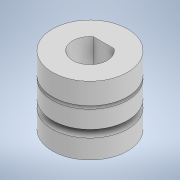
# Autodesk Inventor part: V-Groove Feeder
Saved by Autodesk Inventor 2022.2 (Build 262287000, 287)
## iProperties
Created: 2022-08-20
Part Number: V-Groove Feeder
Material: Generic
Document SubType Name: Modeling
Designer: Ilewicz
Density: 1 g/cm^3
Appearance: Default
Author: Ilewicz
Autodesk Inventor part; units mm, degrees
ref_plane "YZ Plane" through (0, 0, 0) normal (1, 0, 0) x (0, 1, 0)
ref_plane "XZ Plane" through (0, 0, 0) normal (0, 1, 0) x (-1, 0, 0)
ref_plane "XY Plane" through (0, 0, 0) normal (0, 0, 1) x (1, 0, 0)
derived "Motor.ipt"
sketch "Sketch1" plane through (0, 0, 0) normal (0, 1, 0) x (-1, 0, 0)
  circle A0 centre (0, 0) radius 5.5
  circle A1 centre (0, 0) radius 2.525
  line L0 (1.515, -2.02) -> (-1.515, -2.02)
  dimension "d1" = 11
  dimension "d2" = 5.05
  dimension "d3" = 2.02
  constraints: 2 centre point, 2 coincident, 2 end point, 2 point on circle, 1 horizontal
  measures "d1" diameter of A0
  measures "d2" diameter of A1
  measures "d3" distance from line of L0 point (0, 0)
extrude "Extrusion1" add sketch "Sketch1" along normal blind 10 contours A0 | L0 A1 picked at (-0.3501, -2.1121)
sketch "Sketch2" plane through (0, 0, 0) normal (1, 0, 0) x (0, 1, 0)
  line L0 (6.1011, 0) -> (-0.6092, 0)
  line L1 (0, -5.5) -> (10, -5.5) construction
  line L2 (6.8867, -5.5) -> (6.6667, -5.1189)
  line L3 (6.6667, -5.1189) -> (6.4467, -5.5)
  line L4 (3.8833, -5.5) -> (3.3333, -4.5474)
  line L5 (3.3333, -4.5474) -> (2.7833, -5.5)
  line L6 (3.8833, -5.5) -> (2.7833, -5.5)
  line L7 (6.8867, -5.5) -> (6.4467, -5.5)
  line L8 (6.6667, -5.1189) -> (6.6667, -5.5)
  line L9 (3.3333, -4.5474) -> (3.3333, -5.5)
  line L10 (0, 5.5) -> (10, 5.5) projected
  line L11 (5, 5.5) -> (5, -5.5)
  line L12 (0, -5.5) -> (0, 5.5) construction
  line L13 (0, -5.5) -> (0, -4.386) construction
  circle A0 centre (6.6667, -5.5189) radius 0.2 construction
  circle A1 centre (3.3333, -5.5474) radius 0.5 construction
  point P0 (0, 0)
  dimension "d8" = 0.4
  dimension "d9" = 1
  dimension "d10" = 0.44
  dimension "d11" = 1.1
  dimension "d12" = 30
  dimension "d13" = 30
  constraints: 22 end point, 6 point on line, 4 midpoint, 4 tangent, 2 centre point, 2 coincident, 2 horizontal, 2 perpendicular, 1 collinear, 4 other
  measures "d8" diameter of A0
  measures "d9" diameter of A1
  measures "d10" distance of L2.start L3.end
  measures "d11" distance of L4.start L5.end
  measures "d12" angle of L9 L4
  measures "d13" angle of L8 L2
revolve "Revolution1" cut sketch "Sketch2" angle 360 about axis through (0, 6.1011, 0) along (0, -1, 0)
equation "\"d2\" = 1.01 * d_shaft"
equation "\"d3\" = 1.01 * r_flange"
equation "\"d_shaft\" = 5"
equation "\"r_flange\" = 2"
body "Solid1"
